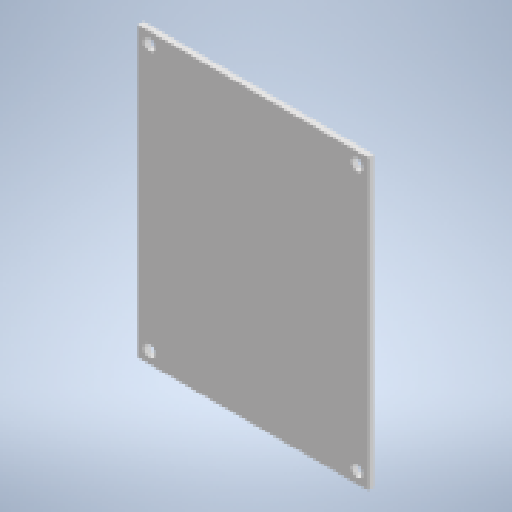
# Autodesk Inventor part: PCB
Saved by Autodesk Inventor 2025.3 (Build 293356000, 356)
## iProperties
Created: 2025-11-23
Part Number: PCB
Material: ABS Plastic
Document SubType Name: Modeling
Designer: Wula
Density: 1.06 g/cm^3
Appearance: Smooth - White
Author: Wula
Autodesk Inventor part; units mm, degrees
ref_plane "YZ Plane" through (0, 0, 0) normal (1, 0, 0) x (0, 1, 0)
ref_plane "XZ Plane" through (0, 0, 0) normal (0, 1, 0) x (-1, 0, 0)
ref_plane "XY Plane" through (0, 0, 0) normal (0, 0, 1) x (1, 0, 0)
sketch "Sketch1" plane through (0, 0, 0) normal (0, 1, 0) x (-1, 0, 0)
  line L0 (-40, 50) -> (40, 50)
  line L1 (40, 50) -> (40, -50)
  line L2 (40, -50) -> (-40, -50)
  line L3 (-40, -50) -> (-40, 50)
  line L4 (-40, 50) -> (40, -50) construction
  line L5 (40, 50) -> (-40, -50) construction
  circle A0 centre (34.29, 45.72) radius 2
  line L6 (-34.29, 45.72) -> (34.29, 45.72) construction
  line L7 (34.29, 45.72) -> (34.29, -45.72) construction
  line L8 (34.29, -45.72) -> (-34.29, -45.72) construction
  line L9 (-34.29, -45.72) -> (-34.29, 45.72) construction
  line L10 (-34.29, 45.72) -> (34.29, -45.72) construction
  line L11 (34.29, 45.72) -> (-34.29, -45.72) construction
  circle A1 centre (34.29, -45.72) radius 2
  circle A2 centre (-34.29, -45.72) radius 2
  circle A3 centre (-34.29, 45.72) radius 2
  point P0 (0, 0)
  dimension "d0" = 100
  dimension "d1" = 80
  dimension "d2" = 4
  dimension "d15" = 91.44
  dimension "d16" = 68.58
  dimension "d17" = 4
  dimension "d18" = 4
  dimension "d19" = 4
  constraints: 24 end point, 4 centre point, 4 coincident, 4 midpoint, 4 parallel, 2 horizontal, 2 perpendicular
  measures "d0" distance of L0.end L1.end
  measures "d1" distance of L0.start L0.end
  measures "d2" diameter of A0
  measures "d15" distance of L6.end L7.end
  measures "d16" distance of L6.start L6.end
  measures "d17" diameter of A1
  measures "d18" diameter of A2
  measures "d19" diameter of A3
extrude "Extrusion1" add sketch "Sketch1" along normal blind 2
body "Solid1"
